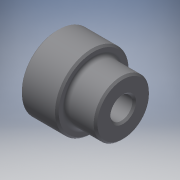
# Autodesk Inventor part: 歯車m2,z18
Saved by Autodesk Inventor 2019.2 (Build 232265000, 265)
## iProperties
Category: PARTsolutions
Company: KHK
Created: 2018-12-15
Part Number: 歯車m2,z18
Material: 一般
Catalog Web Link: www.cadenas.de
Description: Ground Spur Gears (SSG)-
Vendor: KHK
Document SubType Name: Modeling
Designer: psadmin
Manufacturer: KHK
Mass: 32.2448 g
Surface Area: 73.3846 cm^2
Volume: 32.2448 cm^3
Density: 1 g/cm^3
Appearance: PSOLRGB-175-175-175
PSOL_IDENT_0: {$CADENAS_DATA\23d-libs\khk\spur_gears\ground_spur_gears_ssg.prj},174 {VTYP=3D},{NB=SSG2-18},{LINA=S
PSOL_IDENT_1: SG2-18},{NN=Ground Spur Gears (SSG)},{DATE=17.03.2017 04:28:20},{GEOMDATE=10.12.2014 11:17:00},{VERS
PSOL_IDENT_2: ION=},{LINEID=23420},{WBVAR=},{WBNUMERIC=}  {NB=SSG2-18},{LINA=SSG2-18},{KT=DUMMY},{CN=SSG2-18},{M=2
PSOL_IDENT_3: .0},{Z=18},{A=12},{B=30},{C=36.0},{D=40.0},{E=20},{F=16},{G=36},{H=0},{I=0},{K=0},{KD=0.0},{M1=0},{J=
PSOL_IDENT_4: 0.0},{S=S1},{R=2},{N=1},{L=1},{L2=1},{X=1},{M11=0},{XX=0},{HIDE=0},{CBD1=0.0},{CBD2=0.0}
NN: Ground Spur Gears (SSG)
NB: SSG2-18
NBSYN: $CN.
LINA: SSG2-18
CN: SSG2-18
M: 2
Z: 18
A: 12
B: 30
C: 36
D: 40
E: 20
F: 16
G: 36
H: 0
I: 0
K: 0
KD: 0
M1: 0
J: 0
S: S1
SUPPLIER: KHK
ARTICLENO: SSG2-18
BOMINFO: SSG2-18
CREATOR: CADENAS GmbH
Title: SSG2-18
Author: Cadenas PARTsolutions
Autodesk Inventor part; units mm, degrees
ref_plane "YZ Plane" through (0, 0, 0) normal (1, 0, 0) x (0, 1, 0)
ref_plane "XZ Plane" through (0, 0, 0) normal (0, 1, 0) x (-1, 0, 0)
ref_plane "XY Plane" through (0, 0, 0) normal (0, 0, 1) x (1, 0, 0)
sketch "Sketch_8" plane through (0, 0, 0) normal (0, 0, 1) x (1, 0, 0)
  line L0 (36, 0) -> (0, 0)
  line L1 (0, 7) -> (1, 6)
  line L2 (1, 6) -> (35, 6)
  line L3 (35, 6) -> (36, 7)
  line L4 (36, 7) -> (36, 14)
  line L5 (36, 14) -> (35, 15)
  line L6 (35, 15) -> (22, 15)
  arc A0 (20, 17) -> (22, 15) centre (22, 17) ccw
  line L7 (20, 17) -> (20, 19)
  line L8 (20, 19) -> (19, 20)
  line L9 (19, 20) -> (1, 20)
  line L10 (1, 20) -> (0, 19)
  line L11 (0, 19) -> (0, 7)
  constraints: 24 end point, 2 point on circle, 1 centre point
revolve "Revolution1" add sketch "Sketch_8" angle 360 about axis through (36, 0, 0) along (1, 0, 0)
body "Solid1"
